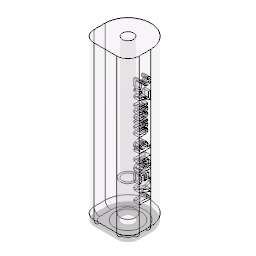
Fiber_Autoclaving_Holder_v9 (Autodesk Fusion 360 design; units mm, degrees)
Autodesk Fusion 360 part; units mm, degrees
sketch "Sketch1" plane through (0, 0, 0) normal (0, 1, 0) x (1, 0, 0)
  circle A0 centre (0, 0) radius 4
  circle A1 centre (0, 0) radius 1.35
  circle A2 centre (0, 0) radius 1
  dimension "d1" = 8
  dimension "d2" = 2.7
  dimension "d3" = 2
  constraint coincident A0.centre A1.centre
  measures "d1" diameter of A0
  measures "d2" diameter of A1
  measures "d3" diameter of A2
extrude "Extrude1" add sketch "Sketch1" along normal blind 28 contours A0 | A1
extrude "Extrude2" cut sketch "Sketch1" along normal blind 6.45 contours A1
fillet "Fillet1" radius 1 1 edges at (-1.2586, 0, 0.4882)
sketch "Sketch2" plane through (0, 28, 0) normal (0, 1, 0) x (-1, 0, 0)
  circle A0 centre (0, 0) radius 1
  circle A1 centre (0, 0) radius 4
  line L0 (0, 0) -> (-4, 0)
  line L1 (0, 0) -> (4, 0)
  line L2 (0, 0) -> (0, 4)
  line L3 (4, 0) -> (0, 0)
  line L4 (0, 0) -> (0, 4)
  line L5 (0, 4) -> (4, 4)
  line L6 (4, 4) -> (4, 0)
  line L7 (0, 4) -> (-4, 4)
  line L8 (-4, 4) -> (-4, 0)
  line L9 (-4, 0) -> (0, 0)
  line L10 (0, 0) -> (0, 4)
  constraint coincident A0.centre A1.centre
  constraint coincident A1 L0.end
  constraint horizontal L0
  constraint coincident A1 L1.end
  constraint parallel L0 L1
  constraint coincident A1 L2.end
  constraint perpendicular L1 L2
  constraint horizontal L3
  constraint vertical L4
  constraint horizontal L5
  constraint vertical L6
  constraint horizontal L7
  constraint vertical L8
  constraint horizontal L9
  constraint vertical L10
extrude "Extrude3" add sketch "Sketch2" against normal up to surface (28 mm away) contours A1 L5 L6 | A1 L7 L8
fillet "Fillet3" radius 2 2 edges at (4, 14, 4) (-4, 14, 4)
fillet "Fillet4" radius 1 6 edges at (4, 0, 1) (0, 0, -4) (-4, 0, 1) (-3.4142, 0, 3.4142) (0, 0, 4) (3.4142, 0, 3.4142)
sketch "Sketch3" plane through (4, 0, 0) normal (1, 0, 0) x (0, 0, -1)
  line L0 (-2, 1) -> (0, 1)
  line L1 (0, 1) -> (0, 28)
  line L2 (0, 28) -> (-2, 28)
  line L3 (-2, 28) -> (-2, 1)
  dimension "d19" = 2
  text T0 "2.7mm d REV1" font "Arial" height 2 bold align centre spacing 1 along the path L3 letters at x, y, angle (0.5293, 24.206, -90) (0.5293, 22.6521, -90) (0.5293, 21.8759, -90) (0.5293, 20.322, -90) (0.5293, 17.8377, -90) (0.5293, 15.3533, -90) (0.5293, 14.5771, -90) (0.5293, 12.8704, -90) (0.5293, 12.0941, -90) (0.5293, 10.0764, -90) (0.5293, 8.2128, -90) (0.5293, 6.3479, -90)
extrude "Extrude4" cut sketch "Sketch3" against normal blind 1 text T0
move_face "OffsetFaces1" [suppressed]
equation "d2 = fiber_hole_diam"
equation "fiber_hole_diam = 2.7 mm"
